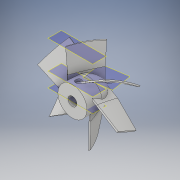
# Autodesk Inventor part: brImp_fan_actual
Saved by Autodesk Inventor 2018 (Build 220112000, 112)
## iProperties
Created: 2018-02-04
Part Number: brImp_fan_actual
Material: Generic
Document SubType Name: Modeling
Designer: Benedikt
Density: 1 g/cm^3
Appearance: Default
Author: Benedikt
## iProperties of the stored document brImp_fan_actual_3DPrint.ipt
Created: 2018-02-05
Part Number: brImp_fan_actual_3DPrint
Material: Generic
Document SubType Name: Modeling
Designer: Benedikt
Density: 1 g/cm^3
Appearance: Default
Author: Benedikt
Autodesk Inventor part; units mm, degrees
ref_plane "YZ Plane" through (0, 0, 0) normal (1, 0, 0) x (0, 1, 0)
ref_plane "XZ Plane" through (0, 0, 0) normal (0, 1, 0) x (-1, 0, 0)
ref_plane "XY Plane" through (0, 0, 0) normal (0, 0, 1) x (1, 0, 0)
sketch "Sketch1" plane through (0, 0, 0) normal (0, 1, 0) x (-1, 0, 0)
  circle A0 centre (0, 0) radius 15.3
  circle A1 centre (0, 0) radius 4.7
  dimension "d0" = 30.6
  dimension "d1" = 9.4
  constraints: 2 centre point, 2 coincident
  measures "d0" diameter of A0
  measures "d1" diameter of A1
extrude "Extrusion1" add sketch "Sketch1" along normal blind 13
sketch "Sketch2" plane through (0, 13, 0) normal (0, 1, 0) x (1, 0, 0)
  line L0 (19.8933, 0) -> (-23.0575, 0) construction
  point P0 (0, 0)
  constraints: 2 end point, 1 horizontal
ref_plane "Work Plane1" through (19.8933, 13, 0) normal (0, 0, -1) x (-1, 0, 0)
sketch "Sketch3" plane through (19.8933, 13, 0) normal (0, 0, -1) x (-1, 0, 0)
  circle A0 centre (19.8933, -6.75) radius 1.95
  line L0 (35.1933, 0) -> (4.5933, 0) projected
  line L1 (15.1933, 0) -> (24.5933, 0) projected
  point P0 (19.8933, -13)
  dimension "d5" = 3.9
  dimension "d18" = 6.75
  constraints: 1 centre point, 1 coincident
  measures "d5" diameter of A0
  measures "d18" distance from line of L1 A0.centre
extrude "Extrusion2" cut sketch "Sketch3" along normal through all both and the other way through all
ref_plane "Work Plane2" through (0, 0, 15.3) normal (0, 0, -1) x (-1, 0, 0)
sketch "Sketch4" plane through (0, 0, 15.3) normal (0, 0, -1) x (-1, 0, 0)
  point P0 (0, 0)
  point P1 (0, 6.35)
  constraints: 1 other
hole "Hole1" at (0, 6.35, 15.3) direction (0, 0, -1) diameter 6.2 depth 6.5 tip angle 118
mirror "Mirror1" about plane through (19.8933, 13, 0) normal (0, 0, -1) of "Hole1"
sketch "Sketch5" plane through (0, 13, 0) normal (0, 1, 0) x (1, 0, 0)
  circle A0 centre (0, 0) radius 15.3 projected
extrude "Extrusion3" add sketch "Sketch5" along normal blind 3
sketch "Sketch6" plane through (19.8933, 13, 0) normal (0, 0, -1) x (-1, 0, 0)
  line L0 (35.1933, 3) -> (4.5933, 3) projected
  line L1 (35.1933, 3) -> (35.1933, 5.6247) construction
  line L2 (35.1933, 5.6247) -> (32.2318, 14.5657) construction
  line L3 (32.2318, 14.5657) -> (19.8933, 23) construction
  spline S0 degree 3 poles (35.1933, 3) (35.1933, 5.6247) (32.2318, 14.5657) (19.8933, 23) knots 1 1 1 1 2 2 2 2
  line L4 (19.8933, 23) -> (19.8933, 3)
  point P0 (19.8933, -13)
  dimension "d20" = 20
  constraints: 2 end point, 1 midpoint, 1 vertical, 3 other
  measures "d20" distance from line of L3.end L0
revolve "Revolution1" add sketch "Sketch6" angle 360 about axis through (0, 36, 0) along (0, -1, 0)
ref_plane "Work Plane3" through (0, 0, 45.3) normal (0, 0, -1) x (-1, 0, 0)
ref_plane "Work Plane4" through (11.0362, 24.8, 15.3) normal (0, 0, -1) x (-0.9892035, -0.1465487, 0)
sketch "Sketch10" plane through (0, 0, 0) normal (0, -1, 0) x (1, 0, 0)
  circle A0 centre (0, 0) radius 4.7 projected
  circle A1 centre (0, 0) radius 42.5
  circle A2 centre (0, 0) radius 150.3264
  dimension "d38" = 85
  constraints: 2 centre point, 2 coincident
  measures "d38" diameter of A1
extrude "Extrusion5" cut sketch "Sketch10" against normal blind 70.75 contours A2
sketch "Sketch13" plane through (11.0362, 24.8, 15.3) normal (0, 0, -1) x (-0.9892035, -0.1465487, 0)
  line L0 (8.8995, 10.5086) -> (18.2823, -2.5987) construction
  line L1 (18.2823, -2.5987) -> (24.7152, -15.0709) construction
  spline S0 degree 2 poles (8.8995, 10.5086) (18.2823, -2.5987) (24.7152, -15.0709) knots 1 1 1 2 2 2
  line L2 (9.9089, 10.9437) -> (19.5369, -1.9769) construction
  line L3 (19.5369, -1.9769) -> (25.8346, -14.1528) construction
  spline S1 degree 2 poles (9.9089, 10.9437) (19.5369, -1.9769) (25.8346, -14.1528) knots 1 1 1 2 2 2
  line L4 (25.8346, -14.1528) -> (24.7152, -15.0709)
  line L5 (9.9089, 10.9437) -> (8.8995, 10.5086)
  point P0 (14.5515, -22.9149)
  constraints: 4 end point, 6 other
sketch "Sketch14" plane through (0, 0, 45.3) normal (0, 0, -1) x (-1, 0, 0)
  line L0 (-5.2132, 30.9665) -> (5.2719, 18.2605) construction
  line L1 (5.2719, 18.2605) -> (12.301, 4.737) construction
  spline S0 degree 2 poles (-5.2132, 30.9665) (5.2719, 18.2605) (12.301, 4.737) knots 1 1 1 2 2 2
  line L2 (-4.4168, 31.9665) -> (5.2719, 20.504) construction
  line L3 (5.2719, 20.504) -> (12.7031, 6.2068) construction
  spline S1 degree 2 poles (-4.4168, 31.9665) (5.2719, 20.504) (12.7031, 6.2068) knots 1 1 1 2 2 2
  line L4 (-4.4168, 31.9665) -> (-5.2132, 30.9665)
  line L5 (12.7031, 6.2068) -> (12.301, 4.737)
  point P0 (0, 0)
  dimension "d66" = 1
  constraints: 4 end point, 6 other
  measures "d66" vertical distance of L2.start L0.start
loft "Loft4" add profiles "Sketch13", "Sketch14"
sketch "Sketch15" plane through (-11.2035, 6.2698, 15.3) normal (0, 0, -1) x (-0.8577707, 0.5140326, 0)
  spline S0 degree 2 poles (0, 0) (2.9359, 13.723) (3.9938, 29.8077) knots 0 0 0 1 1 1 projected
  line L0 (1.4477, 0) -> (0, 0) projected
  spline S1 degree 2 poles (5.0502, 29.5039) (4.3003, 13.4081) (1.4477, 0) knots 0 0 0 1 1 1 projected
  line L1 (3.9938, 29.8077) -> (5.0502, 29.5039) projected
  point P0 (-12.833, 0.3809)
  constraints: 2 other
extrude "Extrusion8" add sketch "Sketch15" along normal blind 14.75
pattern_circular "Circular Pattern4" count 6 over 360 about axis through (0, 0, 0) along (0, 1, 0) of "Loft4", "Extrusion8"
sketch "Sketch12" plane through (0, 0, 0) normal (0, -1, 0) x (1, 0, 0)
  circle A0 centre (0, 0) radius 43
  circle A1 centre (0, 0) radius 65.5972
  dimension "d52" = 86
  constraints: 2 centre point, 2 coincident
  measures "d52" diameter of A0
extrude "Extrusion7" cut sketch "Sketch12" against normal blind 48.25
body "Solid1"
